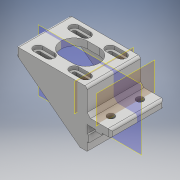
# Autodesk Inventor part: Estrutura - Suporte Z Motor v2
Saved by Autodesk Inventor 2017 (Build 210142000, 142)
## iProperties
Created: 2020-10-04
Part Number: Estrutura - Suporte Z Motor v2
Material: Generic
Document SubType Name: Modeling
Designer: ale
Density: 1 g/cm^3
Appearance: Default
Author: ale
Autodesk Inventor part; units mm, degrees
ref_plane "YZ Plane" through (0, 0, 0) normal (1, 0, 0) x (0, 1, 0)
ref_plane "XZ Plane" through (0, 0, 0) normal (0, 1, 0) x (-1, 0, 0)
ref_plane "XY Plane" through (0, 0, 0) normal (0, 0, 1) x (1, 0, 0)
sketch "Sketch1" plane through (0, 0, 0) normal (0, 0, 1) x (1, 0, 0)
  line L0 (-27.5, 23) -> (27.5, 23)
  line L1 (27.5, 23) -> (27.5, -23)
  line L2 (27.5, -23) -> (-27.5, -23)
  line L3 (-27.5, -23) -> (-27.5, 23)
  line L4 (-27.5, 23) -> (27.5, -23) construction
  line L5 (27.5, 23) -> (-27.5, -23) construction
  point P0 (0, 0)
  dimension "d0" = 55
  dimension "d1" = 46
  constraints: 12 end point, 2 midpoint, 2 parallel, 1 horizontal, 1 perpendicular
  measures "d0" distance of L1.end L2.end
  measures "d1" distance of L0.end L1.end
extrude "Extrusion1" add sketch "Sketch1" along normal blind 6
sketch "Sketch2" plane through (27.5, -23, 0) normal (1, 0, 0) x (0, 0, -1)
  line L0 (-6, 46) -> (-6, 0) projected
  line L1 (-6, 0) -> (16, 0)
  line L2 (16, 0) -> (16, 46)
  line L3 (16, 46) -> (-6, 46)
  line L4 (-6, 46) -> (-6, 0)
  point P0 (0, 23)
  dimension "d4" = 22
  dimension "d5" = 46
  constraints: 8 end point, 2 parallel, 1 horizontal, 1 perpendicular
  measures "d4" distance of L3.end L2.end
  measures "d5" distance of L2.end L1.end
extrude "Extrusion2" add sketch "Sketch2" along normal blind 6
sketch "Sketch4" plane through (27.5, -23, -16) normal (0, 0, -1) x (-1, 0, 0)
  line L0 (0, 0) -> (0, 46) projected
  line L1 (0, 0) -> (-26, 0)
  line L2 (-26, 0) -> (-26, 46)
  line L3 (-26, 46) -> (0, 46)
  line L4 (0, 46) -> (0, 0)
  point P0 (27.5, 23)
  dimension "d8" = 26
  dimension "d35" = 46
  constraints: 8 end point, 2 parallel, 1 horizontal, 1 perpendicular
  measures "d8" distance of L2.end L3.end
  measures "d35" distance between parallel lines of L3 L1
extrude "Extrusion3" add sketch "Sketch4" along normal blind 6
sketch "Sketch5" plane through (27.5, -23, -22) normal (0, 0, -1) x (-1, 0, 0)
  line L0 (0, 46) -> (-26, 46) projected
  line L1 (-6, 0) -> (-26, 0) projected
  line L2 (0, 46) -> (-6, 46)
  line L3 (-6, 46) -> (-6, 0)
  line L4 (-6, 0) -> (0, 0)
  line L5 (0, 0) -> (0, 46)
  point P0 (27.5, 23)
  dimension "d11" = 6
  constraints: 8 end point, 2 parallel, 1 horizontal, 1 perpendicular
  measures "d11" distance of L4.end L1.start
extrude "Extrusion4" add sketch "Sketch5" along normal blind 20
sketch "Sketch6" plane through (27.5, -23, -22) normal (0, 0, -1) x (-1, 0, 0)
  line L0 (-6, 0) -> (-26, 0) projected
  line L1 (-26, 46) -> (-6, 46) projected
  line L2 (-19, 0) -> (-13, 0)
  line L3 (-13, 0) -> (-13, 46)
  line L4 (-13, 46) -> (-19, 46)
  line L5 (-19, 46) -> (-19, 0)
  line L6 (-26, 46) -> (-26, 0) projected
  point P0 (27.5, 23)
  dimension "d14" = 6
  dimension "d15" = 7
  constraints: 8 end point, 2 parallel, 2 point on line, 1 horizontal, 1 perpendicular
  measures "d14" distance of L4.end L3.end
  measures "d15" distance between parallel lines of L6 L5
extrude "Extrusion5" add sketch "Sketch6" along normal blind 1.5 contours L0 L5 L1 L3
sketch "Sketch7" plane through (33.5, -23, -22) normal (1, 0, 0) x (0, 0, -1)
  line L0 (13, 0) -> (7, 0)
  line L1 (7, 0) -> (7, 46)
  line L2 (7, 46) -> (13, 46)
  line L3 (13, 46) -> (13, 0)
  line L4 (20, 46) -> (20, 0) projected
  line L5 (0, 46) -> (20, 46) projected
  point P0 (-22, 23)
  dimension "d18" = 6
  dimension "d19" = 46
  dimension "d20" = 7
  dimension "d36" = 0
  constraints: 8 end point, 2 parallel, 1 horizontal, 1 perpendicular
  measures "d18" distance of L1.end L2.end
  measures "d19" distance of L0.end L1.end
  measures "d20" distance between parallel lines of L4 L3
  measures "d36" distance between parallel lines of L5 L2
extrude "Extrusion6" add sketch "Sketch7" along normal blind 1.5
sketch "Sketch8" plane through (27.5, -23, -23.5) normal (0, 0, -1) x (-1, 0, 0)
  line L0 (-13, 0) -> (-13, 46) projected
  line L1 (-13, 23) -> (-18.895, 23)
  line L2 (-19, 0) -> (-13, 0) projected
  point P0 (27.5, 23)
  point P1 (-16, 10.5)
  point P2 (-16, 35.5)
  dimension "d23" = 10.5
  dimension "d24" = 3
  constraints: 2 end point, 1 horizontal, 1 midpoint, 1 symmetric about line
  measures "d23" distance from line of L2 point (-16, 10.5)
  measures "d24" distance from line of point (-16, 10.5) L0
hole "Hole1" at (43.5, -12.5, -23.5) at (43.5, 12.5, -23.5) direction (0, 0, 1) diameter 6 end through all counterbore diameter 10 counterbore depth 1.5
sketch "Sketch9" plane through (-27.5, -23, 0) normal (0, -1, 0) x (1, 0, 0)
  line L0 (61, -16) -> (61, 6) projected
  line L1 (0, 6) -> (61, 6) projected
  line L2 (61, 6) -> (0, 6)
  line L3 (0, 6) -> (0, 0)
  line L4 (0, 0) -> (54.9849, -42)
  line L5 (55, -42) -> (61, -42) projected
  line L6 (54.9849, -42) -> (61, -42)
  line L7 (61, -42) -> (61, 6)
  point P0 (27.5, 0)
  constraints: 10 end point, 2 perpendicular, 1 horizontal, 1 parallel
extrude "Extrusion7" add sketch "Sketch9" against normal blind 3
ref_plane "Work Plane1" through (-27.5, 0, 6) normal (0, 1, 0) x (1, 0, 0)
mirror "Mirror1" about plane through (-27.5, 0, 6) normal (0, 1, 0) of "Extrusion7"
ref_plane "Work Plane2" through (43.5, -23, 0) normal (1, 0, 0) x (0, 0, -1)
ref_plane "Work Plane3" through (25, -23, 0) normal (1, 0, 0) x (0, 0, -1)
sketch "Sketch11" plane through (27.5, -23, -42) normal (0, 0, -1) x (-1, 0, 0)
  line L0 (0, 3) -> (0, 43) projected
  line L1 (0, 3) -> (-3, 3)
  line L2 (-3, 3) -> (-3, 43)
  line L3 (-3, 43) -> (0, 43)
  line L4 (0, 43) -> (0, 3)
  point P0 (27.5, 23)
  dimension "d39" = 3
  dimension "d40" = 40
  constraints: 8 end point, 2 parallel, 1 horizontal, 1 perpendicular
  measures "d39" distance of L2.end L3.end
  measures "d40" distance of L1.end L2.end
extrude "Extrusion8" cut sketch "Sketch11" against normal blind 42
sketch "Sketch12" plane through (0, 0, 6) normal (0, 0, 1) x (1, 0, 0)
  arc A0 (15, 17.25) -> (15, 13.75) centre (15, 15.5) ccw
  arc A1 (25, 13.75) -> (25, 17.25) centre (25, 15.5) ccw
  line L0 (-27.5, -20) -> (-27.5, 20) projected
  line L1 (-27.5, 0) -> (33.5, 0)
  line L2 (33.5, 23) -> (33.5, -23) projected
  line L3 (-27.5, 23) -> (27.4849, 23) projected
  line L4 (15, 17.25) -> (25, 17.25)
  line L5 (15, 13.75) -> (25, 13.75)
  line L6 (-27.5, -23) -> (33.5, -23) projected
  line L7 (-27.5, 23) -> (33.5, 23) projected
  line L8 (25, 23) -> (25, 0)
  line L9 (25, 16) -> (29.2976, 16)
  line L10 (4.5, 23) -> (4.5, 0)
  arc A2 (-6, 13.75) -> (-6, 17.25) centre (-6, 15.5) ccw
  arc A3 (-16, 17.25) -> (-16, 13.75) centre (-16, 15.5) ccw
  line L11 (-6, 17.25) -> (-16, 17.25)
  line L12 (-6, 13.75) -> (-16, 13.75)
  arc A4 (15, -13.75) -> (15, -17.25) centre (15, -15.5) ccw
  arc A5 (25, -17.25) -> (25, -13.75) centre (25, -15.5) ccw
  line L13 (15, -17.25) -> (25, -17.25)
  line L14 (15, -13.75) -> (25, -13.75)
  arc A6 (-16, -13.75) -> (-16, -17.25) centre (-16, -15.5) ccw
  line L15 (-6, -17.25) -> (-16, -17.25)
  line L16 (-6, -13.75) -> (-16, -13.75)
  arc A7 (-6, -17.25) -> (-6, -13.75) centre (-6, -15.5) ccw
  arc A8 (-0.5, 11.5) -> (-0.5, -11.5) centre (-0.5, 0) ccw
  arc A9 (9.5, -11.5) -> (9.5, 11.5) centre (9.5, 0) ccw
  line L17 (-0.5, 11.5) -> (9.5, 11.5)
  line L18 (9.5, -11.5) -> (-0.5, -11.5)
  point P0 (0, 0)
  point P1 (-16, 16)
  point P2 (25, -16)
  point P3 (-16, -16)
  dimension "d43" = 3.5
  dimension "d44" = 3.5
  dimension "d49" = 8.5
  dimension "d51" = 20.5
  dimension "d52" = 15.5
  dimension "d53" = 23
  dimension "d54" = 23
  dimension "d55" = 5
  dimension "d56" = 5
  constraints: 28 end point, 21 symmetric about line, 20 point on circle, 10 centre point, 7 point on line, 5 tangent, 3 perpendicular, 2 horizontal, 2 midpoint, 6 other
  measures "d43" diameter of A0
  measures "d44" diameter of A1
  measures "d49" distance between parallel lines of L2 L8
  measures "d51" distance between parallel lines of L10 L8
  measures "d52" distance from line of A0.centre L1
  measures "d53" diameter of A8
  measures "d54" diameter of A9
  measures "d55" distance of L10.end A9.centre
  measures "d56" distance of A8.centre L10.end
extrude "Extrusion9" cut sketch "Sketch12" against normal blind 42 contours L4 L8 L5 A0 | A1 L9 L8 | L8 L9 A1 | A9 L18 A8 L1 | L1 L10 L17 A9 | L10 L1 A8 L17 | L12 A3 L11 A2 | L14 A5 L13 A4 | L16 A7 L15 A6
sketch "Sketch14" plane through (0, 0, 6) normal (0, 0, 1) x (1, 0, 0)
  arc A0 (-16, 17.25) -> (-16, 13.75) centre (-16, 15.5) ccw projected
  arc A1 (-16, 19.5) -> (-16, 11.5) centre (-16, 15.5) ccw
  arc A2 (-6, 13.75) -> (-6, 17.25) centre (-6, 15.5) ccw projected
  arc A3 (-6, 11.5) -> (-6, 19.5) centre (-6, 15.5) ccw
  line L0 (-16, 19.5) -> (-6, 19.5)
  line L1 (-6, 11.5) -> (-16, 11.5)
  arc A4 (15, 17.25) -> (15, 13.75) centre (15, 15.5) ccw projected
  arc A5 (15, -13.75) -> (15, -17.25) centre (15, -15.5) ccw projected
  arc A6 (-16, -13.75) -> (-16, -17.25) centre (-16, -15.5) ccw projected
  arc A7 (15, 19.5) -> (15, 11.5) centre (15, 15.5) ccw
  arc A8 (25, 11.5) -> (25, 19.5) centre (25, 15.5) ccw
  line L2 (15, 19.5) -> (25, 19.5)
  line L3 (25, 11.5) -> (15, 11.5)
  arc A9 (15, -11.5) -> (15, -19.5) centre (15, -15.5) ccw
  arc A10 (25, -19.5) -> (25, -11.5) centre (25, -15.5) ccw
  line L4 (15, -11.5) -> (25, -11.5)
  line L5 (25, -19.5) -> (15, -19.5)
  arc A11 (-16, -11.5) -> (-16, -19.5) centre (-16, -15.5) ccw
  arc A12 (-6, -19.5) -> (-6, -11.5) centre (-6, -15.5) ccw
  line L6 (-16, -11.5) -> (-6, -11.5)
  line L7 (-6, -19.5) -> (-16, -19.5)
  point P0 (0, 0)
  dimension "d59" = 8
  dimension "d60" = 8
  dimension "d61" = 8
  dimension "d62" = 8
  dimension "d63" = 8
  dimension "d64" = 8
  dimension "d65" = 8
  dimension "d66" = 8
  constraints: 16 end point, 16 point on circle, 12 tangent, 8 centre point, 5 coincident
  measures "d59" diameter of A1
  measures "d60" diameter of A3
  measures "d61" diameter of A7
  measures "d62" diameter of A8
  measures "d63" diameter of A9
  measures "d64" diameter of A10
  measures "d65" diameter of A11
  measures "d66" diameter of A12
extrude "Extrusion10" cut sketch "Sketch14" against normal blind 3
chamfer "Chamfer1" distance 3 angle 45 1 edges at (33.5, 0, -16)
fillet "Fillet1" radius 2 7 edges at (-27.5, -23, 3) (-27.5, 23, 3) (-27.5, 0, 6) (53.5, 23, -19) (53.5, -23, -19) (33.5, 0, 6) (53.5, 0, -16)
body "Solid1"
